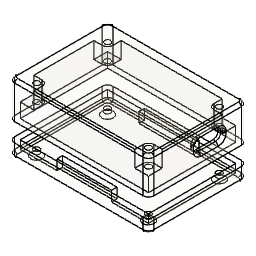
Enclosure (Autodesk Fusion 360 design; units mm, degrees)
Autodesk Fusion 360 part; units mm, degrees
sketch "Sketch1" plane through (0, 0, 0) normal (0, 0, 1) x (1, 0, 0) in component "Enclosure-Bottom"
  line L0 (0, 0) -> (45, 0) construction
  line L1 (45, 0) -> (45, 30) construction
  line L2 (45, 30) -> (0, 30) construction
  line L3 (0, 30) -> (0, 0) construction
  line L4 (-1, -1) -> (46, -1)
  line L5 (46, -1) -> (46, 31)
  line L6 (46, 31) -> (-1, 31)
  line L7 (-1, 31) -> (-1, -1)
  line L8 (-1, -3) -> (46, -3)
  line L9 (48, -1) -> (48, 31)
  line L10 (46, 33) -> (-1, 33)
  line L11 (-3, 31) -> (-3, -1)
  arc A0 (48, 31) -> (46, 33) centre (46, 31) ccw
  arc A1 (-1, 33) -> (-3, 31) centre (-1, 31) ccw
  arc A2 (-3, -1) -> (-1, -3) centre (-1, -1) ccw
  arc A3 (46, -3) -> (48, -1) centre (46, -1) ccw
  dimension "d1" = 45
  dimension "d2" = 30
  dimension "d5" = 1
  dimension "d9" = 2
  dimension "d23" = 3
  dimension "d25" = 3
  dimension "d26" = 3
  dimension "d27" = 3
  constraint horizontal L0
  constraint vertical L1
  constraint horizontal L2
  constraint vertical L3
  constraint coincident L0.start L3.end
  constraint parallel L0 L8
  constraint parallel L1 L9
  constraint parallel L2 L10
  constraint parallel L3 L11
  constraint tangent L9 A0
  constraint tangent L10 A0
  constraint tangent L10 A1
  constraint tangent L11 A1
  constraint equal A0 A1
  constraint tangent L11 A2
  constraint tangent L8 A2
  constraint equal A0 A2
  constraint tangent L8 A3
  constraint tangent L9 A3
  constraint equal A0 A3
  measures "d1" distance of L1.end L2.end
  measures "d2" distance of L0.end L1.end
  measures "d9" radius of A0
  measures "d23" distance of L2 L10
  measures "d25" distance of L0 L8
  measures "d26" distance of L3 L11
  measures "d27" distance of L1 L9
extrude "Extrude1" add sketch "Sketch1" against normal blind 2 contours L4 L5 L6 L7 | L8 L9 L10 L11 A0 A1 A2 A3 makes body 1 in component "Enclosure-Bottom"
extrude "Extrude2" add sketch "Sketch1" along normal blind 3 bodies 1 in component "Enclosure-Bottom"
ref_plane "WorkPlane1" through (22.5, 15, 20) normal (0, 0, 1) x (1, 0, 0)
sketch "Sketch1 (2)" plane through (22.5, 15, 20) normal (0, 0, 1) x (1, 0, 0) in component "Enclosure-Top"
  line L0 (-23.5, -16) -> (23.5, -16)
  line L1 (-23.5, 16) -> (-23.5, -16)
  line L2 (23.5, 16) -> (-23.5, 16)
  line L3 (23.5, -16) -> (23.5, 16)
  line L4 (-23.5, -18) -> (23.5, -18)
  arc A0 (23.5, -18) -> (25.5, -16) centre (23.5, -16) ccw
  line L5 (25.5, -16) -> (25.5, 16)
  line L6 (-25.5, 16) -> (-25.5, -16)
  arc A1 (-25.5, -16) -> (-23.5, -18) centre (-23.5, -16) ccw
  line L7 (23.5, 18) -> (-23.5, 18)
  arc A2 (-23.5, 18) -> (-25.5, 16) centre (-23.5, 16) ccw
  arc A3 (25.5, 16) -> (23.5, 18) centre (23.5, 16) ccw
extrude "Extrude1'" add sketch "Sketch1 (2)" against normal blind 11.25 separate body makes body 2 in component "Enclosure-Top"
extrude "Extrude2'" add sketch "Sketch1 (2)" along normal blind 2 contours L0 L1 L2 L3 | L4 A0 L5 L6 A1 L7 A2 A3 bodies 2 in component "Enclosure-Top"
fillet "Fillet1" radius 1 8 edges at (48, 15, 22) (47.4142, 32.4142, 22) (22.5, 33, 22) (-2.4142, 32.4142, 22) (-3, 15, 22) (-2.4142, -2.4142, 22) (22.5, -3, 22) (47.4142, -2.4142, 22) on bodies 2 in component "Enclosure-Top"
fillet "Fillet1'" radius 1 8 edges at (-3, 15, -2) (-2.4142, 32.4142, -2) (22.5, 33, -2) (47.4142, 32.4142, -2) (48, 15, -2) (47.4142, -2.4142, -2) (22.5, -3, -2) (-2.4142, -2.4142, -2) on bodies 1 in component "Enclosure-Bottom"
sketch "Sketch2" plane through (0, 0, 20) normal (0, 0, -1) x (1, 0, 0) in component "Enclosure-Top"
  line L0 (46, 1) -> (-1, 1)
  line L1 (-1, 1) -> (-1, -31)
  line L2 (-1, -31) -> (46, -31)
  line L3 (46, -31) -> (46, 1)
  line L4 (46, -2) -> (-1, -2) construction
  line L5 (2, 1) -> (2, -31) construction
  line L6 (-1, 1) -> (46, 1)
  line L7 (-1, -31) -> (-1, 1)
  line L8 (46, 1) -> (46, -31)
  line L9 (46, -31) -> (-1, -31)
  line L10 (22.5, 1) -> (22.5, -31) construction
  line L11 (46, -15) -> (-1, -15) construction
  line L12 (46, -28) -> (-1, -28) construction
  line L13 (43, 1) -> (43, -31) construction
  circle A0 centre (43, -2) radius 1.1
  line L14 (43, -4) -> (46, -4)
  line L15 (41, -2) -> (41, 1)
  arc A1 (41, -2) -> (43, -4) centre (43, -2) ccw
  circle A2 centre (2, -2) radius 1.1
  line L16 (4, -2) -> (4, 1)
  arc A3 (2, -4) -> (4, -2) centre (2, -2) ccw
  line L17 (2, -4) -> (-1, -4)
  circle A4 centre (2, -28) radius 1.1
  line L18 (4, -28) -> (4, -31)
  arc A5 (4, -28) -> (2, -26) centre (2, -28) ccw
  line L19 (2, -26) -> (-1, -26)
  line L20 (43, -26) -> (46, -26)
  circle A6 centre (43, -28) radius 1.1
  arc A7 (43, -26) -> (41, -28) centre (43, -28) ccw
  line L21 (41, -28) -> (41, -31)
  dimension "d28" = 3
  dimension "d29" = 3
  dimension "d30" = 2.2
  dimension "d31" = 4
  constraint coincident L3 L4.start
  constraint coincident L1 L4.end
  constraint perpendicular L1 L4
  constraint coincident L0 L5.start
  constraint coincident L2 L5.end
  constraint perpendicular L2 L5
  constraint midpoint L6 L10.start
  constraint midpoint L9 L10.end
  constraint midpoint L8 L11.start
  constraint midpoint L7 L11.end
  constraint symmetric L4.start L11 L12.start
  constraint symmetric L4.end L11 L12.end
  constraint symmetric L5.start L10 L13.start
  constraint symmetric L5.end L10 L13.end
  constraint coincident L13 A0.centre
  constraint coincident L4 A0.centre
  constraint concentric A0 A1
  constraint coincident L13 L14.start
  constraint coincident L8 L14.end
  constraint tangent L14 A1
  constraint coincident L4 L15.start
  constraint coincident L6 L15.end
  constraint tangent L15 A1
  constraint symmetric L10 A0 A2
  constraint symmetric L10 L14.start A3.start
  constraint symmetric L10 L14.end L17.end
  constraint symmetric L10 L15.start L16.start
  constraint symmetric L10 L15.end L16.end
  constraint symmetric L10 A1 A3
  constraint symmetric L11 A0 A6
  constraint symmetric L11 L14.start L20.start
  constraint symmetric L11 L14.end L20.end
  constraint symmetric L11 L15.start A7.end
  constraint symmetric L11 L15.end L21.end
  constraint symmetric L11 A1 A7
  constraint symmetric L11 A2 A4
  constraint symmetric L11 L16.start L18.start
  constraint symmetric L11 L16.end L18.end
  constraint symmetric L11 A3.start A5.end
  constraint symmetric L11 A3 A5
  constraint symmetric L11 L17.end L19.end
  measures "d28" distance of L0 L4
  measures "d29" distance of L5 L7
  measures "d30" diameter of A0
  measures "d31" diameter of A1
extrude "Extrude3" add sketch "Sketch2" along normal blind 6 contours L0 L3 L6 L8 L14 L15 A1 | L0 L1 L6 L7 L16 A3 L17 | L2 L3 L8 L9 L20 A7 L21 | L1 L2 L7 L9 L18 A5 L19 bodies 2 in component "Enclosure-Top"
sketch "Sketch2 (2)" plane through (0, 0, 0) normal (0, 0, 1) x (-1, 0, 0) in component "Enclosure-Bottom"
  line L0 (1, 1) -> (-46, 1)
  line L1 (-46, 1) -> (-46, -31)
  line L2 (-46, -31) -> (1, -31)
  line L3 (1, -31) -> (1, 1)
  line L4 (1, -31) -> (-46, -31)
  line L5 (-46, -31) -> (-46, 1)
  line L6 (1, 1) -> (1, -31)
  line L7 (-46, 1) -> (1, 1)
  line L8 (-12.5, -31) -> (-32.5, -31)
  line L9 (-32.5, -31) -> (-32.5, -29)
  line L10 (-32.5, -29) -> (-12.5, -29)
  line L11 (-12.5, -29) -> (-12.5, -31)
  line L12 (-22.5, -31) -> (-22.5, 1) construction
  line L13 (-46, -15) -> (1, -15) construction
  line L14 (-32.5, -1) -> (-12.5, -1)
  line L15 (-12.5, -1) -> (-12.5, 1)
  line L16 (-32.5, 1) -> (-32.5, -1)
  dimension "d34" = 2
  dimension "d35" = 20
  dimension "d36" = 10
  constraint horizontal L8
  constraint vertical L9
  constraint horizontal L10
  constraint vertical L11
  constraint midpoint L4 L12.start
  constraint midpoint L7 L12.end
  constraint midpoint L5 L13.start
  constraint midpoint L6 L13.end
  constraint coincident L4 L8.end
  constraint symmetric L8.start L13 L15.end
  constraint symmetric L8.end L13 L16.start
  constraint symmetric L9.end L13 L14.start
  constraint symmetric L10.end L13 L14.end
  measures "d34" distance of L8.end L9.end
  measures "d35" distance of L9.end L10.end
  measures "d36" distance of L10.end L12
extrude "Extrude3'" add sketch "Sketch2 (2)" along normal blind 3.75 contours L0 L7 L14 L15 L16 | L2 L4 L8 L9 L10 L11 bodies 1 in component "Enclosure-Bottom"
sketch "Sketch4" plane through (0, 0, -2) normal (0, 0, -1) x (1, 0, 0) in component "Enclosure-Bottom"
  line L0 (-2, 1) -> (-2, -31)
  arc A0 (-2, -31) -> (-1, -32) centre (-1, -31) ccw
  line L1 (-1, -32) -> (46, -32)
  arc A1 (46, -32) -> (47, -31) centre (46, -31) ccw
  line L2 (47, -31) -> (47, 1)
  arc A2 (47, 1) -> (46, 2) centre (46, 1) ccw
  line L3 (46, 2) -> (-1, 2)
  arc A3 (-1, 2) -> (-2, 1) centre (-1, 1) ccw
  circle A4 centre (43, -2) radius 1.1
  circle A5 centre (2, -2) radius 1.1
  circle A6 centre (2, -28) radius 1.1
  circle A7 centre (43, -28) radius 1.1
extrude "Extrude4" cut sketch "Sketch4" against normal up to surface (2 mm away) contours A4 | A5 | A6 | A7 bodies 1 in component "Enclosure-Bottom"
chamfer "Chamfer1" distance 1 angle 45 4 edges at (0.9744, 27.6022, -2) (41.9744, 27.6022, -2) (41.9744, 1.6022, -2) (0.9744, 1.6022, -2) on bodies 1 in component "Enclosure-Bottom"
sketch "Sketch1 (3)" plane through (48, 0, 0) normal (1, 0, 0) x (0, 1, 0)
  line L0 (31, 21) -> (-1, 21)
  line L1 (-1, 21) -> (-1, 8.75)
  line L2 (-1, 8.75) -> (31, 8.75)
  line L3 (31, 8.75) -> (31, 21)
  line L4 (19.025, 14.7) -> (22.665, 14.7)
  arc A0 (22.665, 14.7) -> (24.445, 16.48) centre (22.665, 16.48) ccw
  line L5 (24.445, 16.48) -> (24.445, 17.08)
  arc A1 (24.445, 17.08) -> (22.665, 18.86) centre (22.665, 17.08) ccw
  line L6 (22.665, 18.86) -> (16.285, 18.86)
  arc A2 (16.285, 18.86) -> (14.505, 17.08) centre (16.285, 17.08) ccw
  line L7 (14.505, 17.08) -> (14.505, 16.48)
  arc A3 (14.505, 16.48) -> (16.285, 14.7) centre (16.285, 16.48) ccw
  line L8 (16.285, 14.7) -> (18.975, 14.7)
  line L9 (18.975, 14.7) -> (19.025, 14.7)
  constraint parallel L4 L9
  constraint tangent A1 L6
  constraint tangent L4 A0
  constraint tangent L6 A2
  constraint tangent A2 L7
  constraint tangent A0 L5
  constraint tangent L5 A1
  constraint tangent L7 A3
  constraint tangent A3 L8
extrude "Extrude5" cut sketch "Sketch1 (3)" against normal up to surface (2 mm away) contours L4 A0 L5 A1 L6 A2 L7 A3 L8 L9 sketch seen with x (1, 0, 0) y (0, 1, 0) z (0, 0, 1) at (0, 0, -1) bodies 2 in component "Enclosure-Top"
chamfer "Chamfer2" distance 1 angle 45 8 edges at (48, 15.0263, 14.2213) (48, 14.505, 15.78) (48, 15.0263, 17.3387) (48, 19.475, 17.86) (48, 23.9237, 17.3387) (48, 24.445, 15.78) (48, 23.9237, 14.2213) (48, 19.475, 13.7) on bodies 2 in component "Enclosure-Top"
component "Enclosure-Bottom" placed x (1, 0, 0) y (0, 1, 0) z (0, 0, 1) at (0, 0, 0)
component "Enclosure-Top" placed x (1, 0, 0) y (0, 1, 0) z (0, 0, 1) at (0, 0, 1)
equation "d1 = length"
equation "d2 = width"
equation "wall_thickness = 2 mm"
equation "margin = 1 mm"
equation "d5 = margin"
equation "fillet_radius = 2 mm"
equation "height = 15 mm"
equation "d9 = fillet_radius"
equation "d10 = -wall_thickness"
equation "d12 = height / 5"
equation "d14 = height + wall_thickness"
equation "d15 = -height * ( 3 / 4 )"
equation "d17 = wall_thickness"
equation "d20 = 0.5 * fillet_radius"
equation "d22 = 0.5 * fillet_radius"
equation "d23 = wall_thickness + margin"
equation "d25 = wall_thickness + margin"
equation "d26 = wall_thickness + margin"
equation "d27 = wall_thickness + margin"
equation "d28 = 2 mm + margin"
equation "d29 = 2 mm + margin"
equation "d32 = height / 2.5"
equation "d34 = wall_thickness"
equation "d35 = 10 * wall_thickness"
equation "d36 = ( 10 * wall_thickness ) / 2"
equation "d37 = height / 4"
equation "length = 45 mm"
equation "width = 30 mm"
